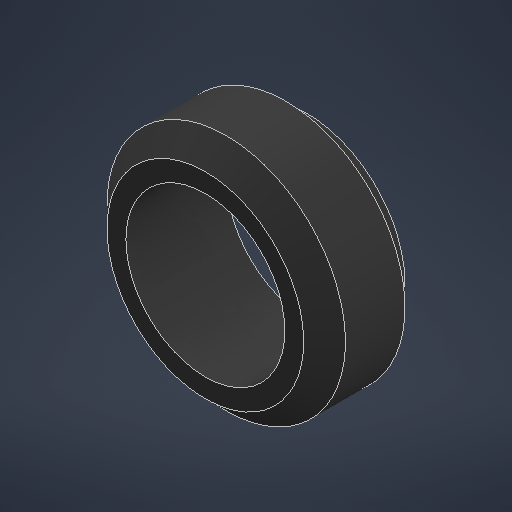
# Autodesk Inventor part: Rueda v
Saved by Autodesk Inventor 2026 (Build 300175050, 175E)
## iProperties
Created: 2025-07-17
Part Number: Rueda v
Material: Caucho
Document SubType Name: Modeling
Designer: bello
Density: 0.93 g/cm^3
Appearance: Caucho - Negro
Author: bello
Autodesk Inventor part; units mm, degrees
ref_plane "YZ Plane" through (0, 0, 0) normal (1, 0, 0) x (0, 1, 0)
ref_plane "XZ Plane" through (0, 0, 0) normal (0, 1, 0) x (-1, 0, 0)
ref_plane "XY Plane" through (0, 0, 0) normal (0, 0, 1) x (1, 0, 0)
sketch "Boceto2" plane through (0, 0, 0) normal (1, 0, 0) x (0, 1, 0)
  line L0 (8, 5.1) -> (8, 0)
  line L1 (8, 0) -> (8, -5.1)
  line L2 (8, -5.1) -> (9.9, -5.1)
  line L3 (9.9, -5.1) -> (12, -3)
  line L4 (12, -3) -> (12, 3)
  line L5 (12, 3) -> (9.9, 5.1)
  line L6 (9.9, 5.1) -> (8, 5.1)
  line L7 (0, 19.536) -> (0, -22.6626)
  point P0 (0, 0)
  dimension "d2" = 6
  dimension "d3" = 5.1
  dimension "d4" = 4
  dimension "d5" = 135
  dimension "d6" = 5.1
  dimension "d7" = 8
  constraints: 16 end point, 3 equal length, 2 parallel, 2 perpendicular, 2 vertical, 1 point on line
  measures "d2" distance of L3.end L4.end
  measures "d3" distance of L0.start L0.end
  measures "d4" distance between parallel lines of L0 L4
  measures "d5" angle of L6 L5
  measures "d6" distance from line of point (0, 0) L2
  measures "d7" distance from line of point (0, 0) L1
revolve "Revolución1" add sketch "Boceto2" angle 360 about axis through (0, 0, 19.536) along (0, 0, -1)
